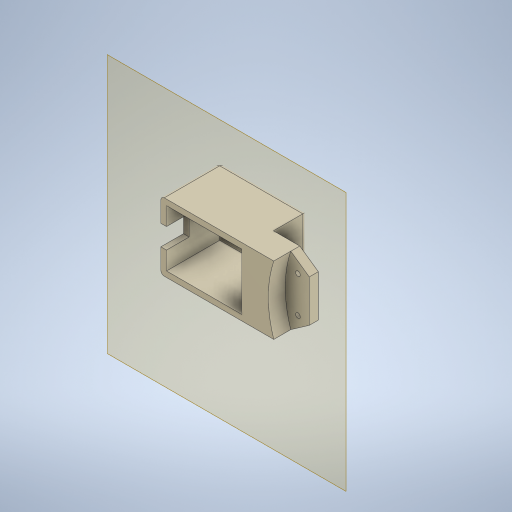
# Autodesk Inventor part: base-stepper-holder
Saved by Autodesk Inventor 2024 (Build 280153000, 153)
## iProperties
Created: 2024-02-17
Part Number: base-stepper-holder
Material: Generic
Document SubType Name: Modeling
Designer: MaartenGeorgesBuelen
Density: 1 g/cm^3
Appearance: Default
Author: MaartenGeorgesBuelen
## iProperties of the stored document base-stepper-holder_3DPrint.ipt
Created: 2024-03-06
Part Number: base-stepper-holder_3DPrint
Material: Generic
Document SubType Name: Modeling
Designer: MaartenGeorgesBuelen
Density: 1 g/cm^3
Appearance: Default
Author: MaartenGeorgesBuelen
Autodesk Inventor part; units mm, degrees
ref_plane "YZ Plane" through (0, 0, 0) normal (1, 0, 0) x (0, 1, 0)
ref_plane "XZ Plane" through (0, 0, 0) normal (0, 1, 0) x (-1, 0, 0)
ref_plane "Work Plane1" through (-132.9045, 0, 0) normal (0, 0, 1) x (1, 0, 0)
ref_plane "Work Plane2" through (-110.9217, -110.9217, -15) normal (0, 0, -1) x (0, 1, 0)
sketch "Sketch1" plane through (-132.9045, 0, 0) normal (0, 0, 1) x (1, 0, 0)
  arc A0 (116.9045, 94.6573) -> (116.9045, -94.6573) centre (132.9045, 0) ccw projected
  arc A1 (116.9045, -94.6573) -> (131.4538, -104) centre (131.4538, -88) ccw projected
  line L0 (131.4538, -104) -> (134.3553, -104) projected
  arc A2 (134.3553, -104) -> (148.9045, -94.6573) centre (134.3553, -88) ccw projected
  arc A3 (148.9045, -94.6573) -> (206.8801, -61.185) centre (132.9045, 0) ccw projected
  arc A4 (206.8801, -61.185) -> (222.2458, -53.2564) centre (208.3894, -45.2564) ccw projected
  line L1 (222.2458, -53.2564) -> (223.6965, -50.7436) projected
  arc A5 (223.6965, -50.7436) -> (222.8801, -33.4722) centre (209.8401, -42.7436) ccw projected
  arc A6 (222.8801, -33.4722) -> (222.8801, 33.4722) centre (132.9045, 0) ccw projected
  arc A7 (222.8801, 33.4722) -> (223.6965, 50.7436) centre (209.8401, 42.7436) ccw projected
  line L2 (223.6965, 50.7436) -> (222.2458, 53.2564) projected
  arc A8 (222.2458, 53.2564) -> (206.8801, 61.185) centre (208.3894, 45.2564) ccw projected
  arc A9 (206.8801, 61.185) -> (148.9045, 94.6573) centre (132.9045, 0) ccw projected
  arc A10 (148.9045, 94.6573) -> (134.3553, 104) centre (134.3553, 88) ccw projected
  line L3 (134.3553, 104) -> (131.4538, 104) projected
  arc A11 (131.4538, 104) -> (116.9045, 94.6573) centre (131.4538, 88) ccw projected
  circle A12 centre (132.9045, 0) radius 3.5 projected
  circle A13 centre (132.9045, -100) radius 3 projected
  circle A14 centre (63.6225, -40) radius 3.5 projected
  circle A15 centre (132.9045, -80) radius 3.5 projected
  circle A16 centre (202.1866, -40) radius 3.5 projected
  circle A17 centre (202.1866, 40) radius 3.5 projected
  circle A18 centre (132.9045, 80) radius 3.5 projected
  circle A19 centre (63.6225, 40) radius 3.5 projected
  circle A20 centre (219.5071, -50) radius 3 projected
  circle A21 centre (219.5071, 50) radius 3 projected
  circle A22 centre (132.9045, 100) radius 3 projected
  line L4 (36.9045, 0) -> (36.9045, 30)
  line L5 (36.9045, 30) -> (41.7124, 30)
  line L6 (36.9045, 0) -> (36.9045, -30)
  line L7 (36.9045, -30) -> (41.7124, -30)
  line L8 (36.9045, 30) -> (-58.0955, 30)
  line L9 (-58.0955, 30) -> (-58.0955, -30)
  line L10 (-58.0955, -30) -> (36.9045, -30)
  line L11 (36.9045, -30) -> (36.9045, 30)
  circle A23 centre (48.0955, -16) radius 2.1 projected
  circle A24 centre (48.0955, 16) radius 2.1 projected
  point P0 (132.9045, 0)
  dimension "d0" = 30
  dimension "d1" = 30
  dimension "d2" = 95
  dimension "d3" = 60
  constraints: 16 end point, 3 perpendicular, 3 point on circle, 2 parallel, 1 horizontal, 1 point on line, 1 tangent, 1 vertical
  measures "d0" distance of L4.start L4.end
  measures "d1" distance of L4.start L6.end
  measures "d2" distance of L10.end L9.end
  measures "d3" distance of L9.end L8.end
extrude "Extrusion1" add sketch "Sketch1" against normal up to surface (15 mm away) contours A0 L4 L5 | L6 L10 L9 L8 L4 | A0 L7 L6
sketch "Sketch2" plane through (-91.1921, 30, -15) normal (0, 0, -1) x (-1, 0, 0)
  circle A0 centre (-91.1921, -30) radius 3.5 projected
  arc A1 (-91.1921, 66) -> (-174.3305, 18) centre (-91.1921, -30) ccw projected
  circle A2 centre (-160.4741, 10) radius 16 projected
  arc A3 (-174.3305, 18) -> (-174.3305, -78) centre (-91.1921, -30) ccw projected
  circle A4 centre (-160.4741, -70) radius 16 projected
  arc A5 (-174.3305, -78) -> (-91.1921, -126) centre (-91.1921, -30) ccw projected
  circle A6 centre (-91.1921, -110) radius 16 projected
  arc A7 (-91.1921, -126) -> (-8.0537, -78) centre (-91.1921, -30) ccw projected
  circle A8 centre (-21.9101, -70) radius 16 projected
  arc A9 (-8.0537, -78) -> (-8.0537, 18) centre (-91.1921, -30) ccw projected
  circle A10 centre (-21.9101, 10) radius 16 projected
  arc A11 (-8.0537, 18) -> (-91.1921, 66) centre (-91.1921, -30) ccw projected
  circle A12 centre (-91.1921, 50) radius 16 projected
  line L0 (99.8079, 0) -> (99.8079, -60) projected
  line L1 (0, 0) -> (99.8079, 0) projected
  arc A13 (0, -60) -> (0, 0) centre (-91.1921, -30) ccw projected
  line L2 (99.8079, -60) -> (0, -60) projected
  circle A14 centre (-6.383, -14) radius 2.1
  line L3 (0, 0) -> (-16.383, -11.4715)
  line L4 (0, 0) -> (20, 0) construction
  line L5 (0, -60) -> (-16.383, -48.5285)
  line L6 (0, -60) -> (20, -60) construction
  line L7 (99.8079, -60) -> (0, -60) projected
  line L8 (-16.383, -48.5285) -> (-16.383, -11.4715)
  circle A15 centre (-6.383, -46) radius 2.1
  circle A16 centre (-6.383, -46) radius 2.1 projected
  circle A17 centre (-6.383, -14) radius 2.1 projected
  point P0 (-91.1921, -30)
  dimension "d6" = 4.2
  dimension "d7" = 14
  dimension "d8" = 20
  dimension "d9" = 145
  dimension "d10" = 20
  dimension "d11" = 145
  dimension "d12" = 10
  dimension "d13" = 14
  dimension "d14" = 10
  constraints: 10 end point, 2 centre point, 2 equal length, 2 horizontal, 2 vertical alignment, 1 equal radius, 4 other
  measures "d6" diameter of A14
  measures "d7" distance from line of L1 A14.centre
  measures "d8" distance of L1.start L3.end
  measures "d9" angle of L3 L4
  measures "d10" distance of L2.end L5.end
  measures "d11" angle of L6 L5
  measures "d12" distance from line of L8 A14.centre
  measures "d13" distance from line of L2 A15.centre
  measures "d14" distance from line of L8 A15.centre
extrude "Extrusion2" add sketch "Sketch2" along normal blind 8 contours L1 L0 L2 A9 | A9 L5 L8 L3
sketch "Sketch3" plane through (-91.1921, 30, -23) normal (0, 0, -1) x (-1, 0, 0)
  line L0 (38.3079, -51.5) -> (81.3079, -51.5)
  line L1 (81.3079, -51.5) -> (81.3079, -8.5)
  line L2 (81.3079, -8.5) -> (38.3079, -8.5)
  line L3 (38.3079, -8.5) -> (38.3079, -51.5)
  line L4 (38.3079, -51.5) -> (81.3079, -8.5) construction
  line L5 (81.3079, -51.5) -> (38.3079, -8.5) construction
  line L6 (99.8079, -60) -> (99.8079, 0) projected
  line L7 (99.8079, 0) -> (0, 0) projected
  line L8 (99.8079, -60) -> (0, -60) projected
  line L9 (99.8079, 0) -> (23.3079, 0)
  line L10 (23.3079, 0) -> (23.3079, -60)
  line L11 (23.3079, -60) -> (99.8079, -60)
  line L12 (99.8079, -60) -> (99.8079, 0)
  line L13 (28.3079, -55) -> (28.3079, -5)
  line L14 (28.3079, -5) -> (94.8079, -5)
  line L15 (94.8079, -5) -> (94.8079, -55)
  line L16 (94.8079, -55) -> (28.3079, -55)
  point P0 (-91.1921, -30)
  point P1 (59.8079, -30)
  point P2 (23.3079, 0)
  dimension "d17" = 43
  dimension "d18" = 43
  dimension "d26" = 30
  dimension "d29" = 40
  dimension "d30" = 15
  dimension "d31" = 5
  constraints: 28 end point, 6 parallel, 3 perpendicular, 2 horizontal, 2 midpoint, 1 point on line, 3 other
  measures "d17" distance of L2.end L1.end
  measures "d18" distance of L1.end L0.end
  measures "d26" distance from line of L7 point (59.808, -30)
  measures "d29" distance from line of L6 point (59.808, -30)
  measures "d30" distance between parallel lines of L10 L3
  measures "d31" distance between parallel lines of L10 L13
extrude "Extrusion3" add sketch "Sketch3" along normal blind 24 contours L8 L10 L7 L6
sketch "Sketch4" plane through (-91.1921, 30, -47) normal (0, 0, -1) x (-1, 0, 0)
  circle A0 centre (41.8079, -14.5) radius 1.5 projected
  circle A1 centre (41.8079, -45.5) radius 1.5 projected
  circle A2 centre (72.8079, -14.5) radius 1.5 projected
  circle A3 centre (72.8079, -45.5) radius 1.5 projected
  circle A4 centre (57.3079, -30) radius 11 projected
  line L0 (76.3079, -9) -> (78.3079, -11) projected
  line L1 (76.3079, -9) -> (38.3079, -9) projected
  line L2 (36.3079, -11) -> (38.3079, -9) projected
  line L3 (36.3079, -11) -> (36.3079, -49) projected
  line L4 (38.3079, -51) -> (36.3079, -49) projected
  line L5 (38.3079, -51) -> (76.3079, -51) projected
  line L6 (78.3079, -49) -> (76.3079, -51) projected
  line L7 (78.3079, -49) -> (78.3079, -11) projected
  line L8 (23.3079, -60) -> (99.8079, -60) projected
  line L9 (99.8079, -60) -> (99.8079, 0) projected
  line L10 (99.8079, 0) -> (23.3079, 0) projected
  line L11 (23.3079, 0) -> (23.3079, -60) projected
  line L12 (28.3079, -55) -> (28.3079, -5) projected
  line L13 (28.3079, -5) -> (94.8079, -5) projected
  line L14 (94.8079, -5) -> (94.8079, -55) projected
  line L15 (94.8079, -55) -> (28.3079, -55) projected
  point P0 (-91.1921, -30)
extrude "Extrusion4" cut sketch "Sketch4" against normal through all contours A1 | A2 | A3 | A4
sketch "Sketch5" plane through (-91.1921, 30, -23) normal (0, 0, -1) x (-1, 0, 0)
  circle A0 centre (41.8079, -45.5) radius 1.5 projected
  circle A1 centre (57.3079, -30) radius 11 projected
  circle A2 centre (72.8079, -45.5) radius 1.5 projected
  circle A3 centre (72.8079, -14.5) radius 1.5 projected
  line L0 (28.3079, -55) -> (94.8079, -55) projected
  line L1 (94.8079, -55) -> (94.8079, -5) projected
  line L2 (94.8079, -5) -> (28.3079, -5) projected
  line L3 (28.3079, -5) -> (28.3079, -55) projected
  point P0 (-91.1921, -30)
extrude "Extrusion5" cut sketch "Sketch5" against normal through all
sketch "Sketch6" plane through (-91.1921, 30, -47) normal (0, 0, -1) x (-1, 0, 0)
  line L0 (23.3079, -60) -> (99.8079, -60) projected
  line L1 (99.8079, -60) -> (99.8079, 0) projected
  line L2 (99.8079, 0) -> (23.3079, 0) projected
  line L3 (23.3079, 0) -> (23.3079, -60) projected
  line L4 (28.3079, -55) -> (28.3079, -5) projected
  line L5 (28.3079, -5) -> (94.8079, -5) projected
  line L6 (94.8079, -5) -> (94.8079, -55) projected
  line L7 (94.8079, -55) -> (28.3079, -55) projected
  circle A0 centre (41.8079, -14.5) radius 1.5 projected
  circle A1 centre (72.8079, -14.5) radius 1.5 projected
  circle A2 centre (72.8079, -45.5) radius 1.5 projected
  circle A3 centre (41.8079, -45.5) radius 1.5 projected
  circle A4 centre (41.8079, -14.5) radius 1.7
  circle A5 centre (72.8079, -14.5) radius 1.7
  circle A6 centre (72.8079, -45.5) radius 1.7
  circle A7 centre (41.8079, -45.5) radius 1.7
  line L8 (41.8079, -43.8) -> (72.8079, -43.8)
  line L9 (72.8079, -47.2) -> (41.8079, -47.2)
  line L10 (41.8079, -12.8) -> (72.8079, -12.8)
  line L11 (72.8079, -16.2) -> (41.8079, -16.2)
  line L12 (41.8079, -16.2) -> (28.3079, -16.2)
  line L13 (41.8079, -12.8) -> (28.3079, -12.8)
  line L14 (72.8079, -12.8) -> (94.8079, -12.8)
  line L15 (72.8079, -16.2) -> (94.8079, -16.2)
  line L16 (72.8079, -43.8) -> (94.8079, -43.8)
  line L17 (72.8079, -47.2) -> (94.8079, -47.2)
  line L18 (41.8079, -47.2) -> (28.3079, -47.2)
  line L19 (41.8079, -43.8) -> (28.3079, -43.8)
  circle A8 centre (57.3079, -30) radius 11 projected
  circle A9 centre (57.3079, -30) radius 11.5
  line L20 (57.3079, -18.5) -> (28.3079, -18.5)
  line L21 (57.3079, -18.5) -> (94.8079, -18.5)
  line L22 (57.3079, -41.5) -> (94.8079, -41.5)
  line L23 (57.3079, -41.5) -> (28.3079, -41)
  point P0 (-91.1921, -30)
  point P1 (56.9115, -41.4932)
  dimension "d32" = 0.2
  dimension "d33" = 0.2
  dimension "d34" = 0.2
  dimension "d35" = 0.2
  dimension "d39" = 0.5
  constraints: 32 end point, 21 point on line, 10 point on circle, 7 tangent, 5 centre point, 2 parallel, 1 horizontal, 1 perpendicular
  measures "d32" radial gap between concentric circles of A0 A4
  measures "d33" radial gap between concentric circles of A1 A5
  measures "d34" radial gap between concentric circles of A2 A6
  measures "d35" radial gap between concentric circles of A3 A7
  measures "d39" radial gap between concentric circles of A8 A9
extrude "Extrusion6" add sketch "Sketch6" along normal blind 5 contours L3 L2 L1 L0 | L4 L18 L9 L17 L6 L7 | L4 L23 L22 L6 L16 L8 L19 | L4 L12 L11 L15 L6 L21 L20 | L4 L5 L6 L14 L10 L13
fillet "Fillet1" radius 3 7 edges at (-114.5, -30, -37.5) (-152.75, -30, -52) (-114.5, 0, -52) (-152.75, 30, -52) (-191, -30, -26) (-191, 0, -52) (-191, 30, -26)
sketch "Sketch7" plane through (-191, -27, 0) normal (-1, 0, 0) x (0, 0, 1)
  line L0 (0, 27) -> (-20, 27)
  line L1 (-20, 27) -> (-20, 17.9937)
  line L2 (-20, 17.9937) -> (0, 17.9937)
  line L3 (0, 17.9937) -> (0, 27)
  line L4 (0, 27) -> (-20, 27)
  line L5 (-20, 27) -> (-20, 35.9937)
  line L6 (-20, 35.9937) -> (0, 35.9937)
  line L7 (0, 35.9937) -> (0, 27)
  dimension "d41" = 20
  dimension "d42" = 18
  constraints: 16 end point, 4 parallel, 2 horizontal, 2 perpendicular, 1 point on line
  measures "d41" distance of L5.end L6.end
  measures "d42" distance between parallel lines of L6 L2
extrude "Extrusion7" cut sketch "Sketch7" against normal up to surface (5 mm away)
body "Solid1"
